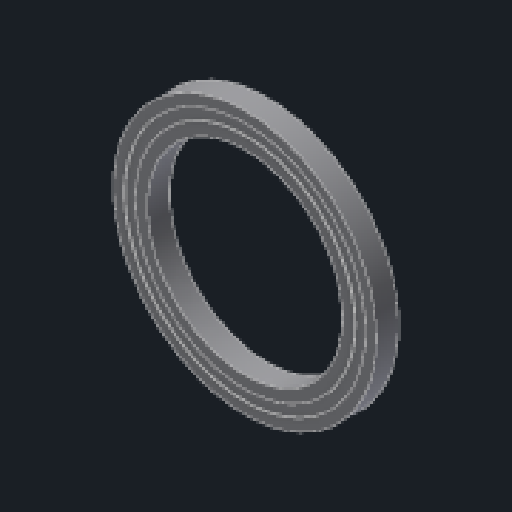
# Autodesk Inventor part: TorsoEncoderAlignmentRing
Saved by Autodesk Inventor 2025.2 (Build 292293000, 293)
## iProperties
Created: 2025-09-22
Part Number: TorsoEncoderAlignmentRing
Material: Generic
Document SubType Name: Modeling
Designer: valer
Density: 1 g/cm^3
Appearance: Default
Author: valer
Autodesk Inventor part; units mm, degrees
ref_plane "YZ Plane" through (0, 0, 0) normal (1, 0, 0) x (0, 1, 0)
ref_plane "XZ Plane" through (0, 0, 0) normal (0, 1, 0) x (-1, 0, 0)
ref_plane "XY Plane" through (0, 0, 0) normal (0, 0, 1) x (1, 0, 0)
sketch "Base" plane through (0, 0, 0) normal (0, 0, 1) x (1, 0, 0)
  circle A0 centre (0, 0) radius 61
  circle A1 centre (0, 0) radius 45.25
  dimension "d0" = 122
  dimension "d1" = 90.5
  constraints: 2 centre point, 2 coincident
  measures "d0" diameter of A0
  measures "d1" diameter of A1
extrude "BaseFeature" add sketch "Base" along normal blind 10.33
sketch "Sketch2" plane through (0, 0, 10.33) normal (0, 0, 1) x (1, 0, 0)
  circle A0 centre (0, 0) radius 55.9435 projected
  circle A1 centre (0, 0) radius 50.8 projected
  point P0 (0, 0)
extrude "Extrusion2" cut sketch "Sketch2" against normal blind 0.5
sketch "Sketch4" plane through (0, 0, 0) normal (0, 0, -1) x (-1, 0, 0)
  circle A0 centre (-40.3005, 39.242) radius 2.75 projected
  circle A1 centre (-0.7484, 56.245) radius 2.75 projected
  circle A2 centre (39.242, 40.3005) radius 2.75 projected
  circle A3 centre (-56.245, -0.7484) radius 2.75 projected
  circle A4 centre (-39.242, -40.3005) radius 2.75 projected
  circle A5 centre (56.245, 0.7484) radius 2.75 projected
  circle A6 centre (0.7484, -56.245) radius 2.75 projected
  circle A7 centre (40.3005, -39.242) radius 2.75 projected
  point P0 (0, 0)
extrude "Extrusion3" cut sketch "Sketch4" against normal through all
sketch "Sketch5" plane through (0, 0, 10.33) normal (0, 0, 1) x (1, 0, 0)
  arc A0 (-38.1325, -40.9339) -> (-41.9341, -37.0298) centre (-40.3005, -39.242) ccw projected
  arc A1 (-55.9084, -1.9809) -> (-55.8359, 3.4678) centre (-56.245, 0.7484) ccw projected
  arc A2 (-40.9339, 38.1325) -> (-37.0298, 41.9341) centre (-39.242, 40.3005) ccw projected
  arc A3 (-1.9809, 55.9084) -> (3.4678, 55.8359) centre (0.7484, 56.245) ccw projected
  arc A4 (38.1325, 40.9339) -> (41.9341, 37.0298) centre (40.3005, 39.242) ccw projected
  arc A5 (55.9084, 1.9809) -> (55.8359, -3.4678) centre (56.245, -0.7484) ccw projected
  arc A6 (40.9339, -38.1325) -> (37.0298, -41.9341) centre (39.242, -40.3005) ccw projected
  arc A7 (1.9809, -55.9084) -> (-3.4678, -55.8359) centre (-0.7484, -56.245) ccw projected
  arc A8 (-41.9341, -37.0298) -> (-38.1325, -40.9339) centre (-40.3005, -39.242) ccw projected
  circle A9 centre (-40.3005, -39.242) radius 5.25
  arc A10 (-55.8359, 3.4678) -> (-55.9084, -1.9809) centre (-56.245, 0.7484) ccw projected
  circle A11 centre (-56.245, 0.7484) radius 5.25
  circle A12 centre (-39.242, 40.3005) radius 5.25
  circle A13 centre (0.7484, 56.245) radius 5.25
  circle A14 centre (40.3005, 39.242) radius 5.25
  circle A15 centre (56.245, -0.7484) radius 5.25
  arc A16 (37.0298, -41.9341) -> (40.9339, -38.1325) centre (39.242, -40.3005) ccw projected
  circle A17 centre (39.242, -40.3005) radius 5.25
  arc A18 (-3.4678, -55.8359) -> (1.9809, -55.9084) centre (-0.7484, -56.245) ccw projected
  circle A19 centre (-0.7484, -56.245) radius 5.25
  point P0 (0, 0)
  dimension "d8" = 10.5
  constraints: 8 centre point, 8 coincident, 7 equal radius
  measures "d8" diameter of A9
extrude "Extrusion4" cut sketch "Sketch5" against normal blind 6.5 contours A8 A0 | A10 A1 | A16 A6 | A18 A7 | A9 | A11 | A12 | A13 | A14 | A15 | A17 | A19
fillet "Fillet1" radius 2 16 edges at (44.1928, -42.0476, 7.08) (40.8568, -45.296, 7.08) (60.9192, -3.139, 7.08) (60.9811, 1.5169, 7.08) (42.0476, 44.1928, 7.08) (45.296, 40.8568, 7.08) (-1.5169, 60.9811, 7.08) (3.139, 60.9192, 7.08) (-44.1928, 42.0476, 7.08) (-40.8568, 45.296, 7.08) (-60.9811, -1.5169, 7.08) (-60.9192, 3.139, 7.08) (-42.0476, -44.1928, 7.08) (-45.296, -40.8568, 7.08) (1.5169, -60.9811, 7.08) (-3.139, -60.9192, 7.08)
body "Solid1"
